# Autodesk Inventor part: SupportBase
Saved by Autodesk Inventor 2014 SP1 (Build 180222100, 222)
## iProperties
Created: 2017-05-14
Part Number: SupportBase
Material: Generic
Document SubType Name: Modeling
Designer: danielsikar
Density: 1 g/cm^3
Appearance: Default
Author: danielsikar
Autodesk Inventor part; units mm, degrees
ref_plane "YZ Plane" through (0, 0, 0) normal (1, 0, 0) x (0, 1, 0)
ref_plane "XZ Plane" through (0, 0, 0) normal (0, 1, 0) x (-1, 0, 0)
ref_plane "XY Plane" through (0, 0, 0) normal (0, 0, 1) x (1, 0, 0)
ref_plane "Work Plane1" through (-57.455, -3.5, -14.8) normal (0, 0, 1) x (0, 1, 0)
ref_plane "Work Plane2" through (-57.455, -3.5, -14.8) normal (0, 0, 1) x (0, 1, 0)
ref_plane "Work Plane3" through (-17.4, -11.75, -16.8) normal (1, 0, 0) x (0, 0, -1)
sketch "Sketch3" plane through (-17.4, -11.75, -16.8) normal (1, 0, 0) x (0, 0, -1)
  line L0 (-2, 0) -> (2, 0) construction
  line L1 (-2, 0) -> (-2, -28.25) construction
  line L2 (2, -28.25) -> (-2, -28.25) construction
  line L3 (2, 0) -> (2, -28.25) construction
  line L4 (2, -28.25) -> (-2, -28.25) construction
  line L5 (-2, -28.25) -> (-2, -19.25) construction
  line L6 (-2, -19.25) -> (2, -19.25) construction
  line L7 (2, -19.25) -> (2, -28.25) construction
  line L8 (2, -28.25) -> (-2, -28.25)
  line L9 (-2, -28.25) -> (-2, -19.25)
  line L10 (-2, -19.25) -> (2, -19.25)
  line L11 (2, -19.25) -> (2, -28.25)
  point P0 (-16.8, 11.75)
  dimension "d0" = 4
  dimension "d1" = 9
  dimension "d2" = 4
  dimension "d3" = 9
  constraints: 16 end point, 4 parallel, 2 horizontal, 2 perpendicular
  measures "d0" distance of L5.end L6.end
  measures "d1" distance of L4.end L5.end
  measures "d2" distance of L5.end L10.end
  measures "d3" distance of L8.end L5.end
extrude "Extrusion1" add sketch "Sketch3" along normal blind 5
body "Solid1"
